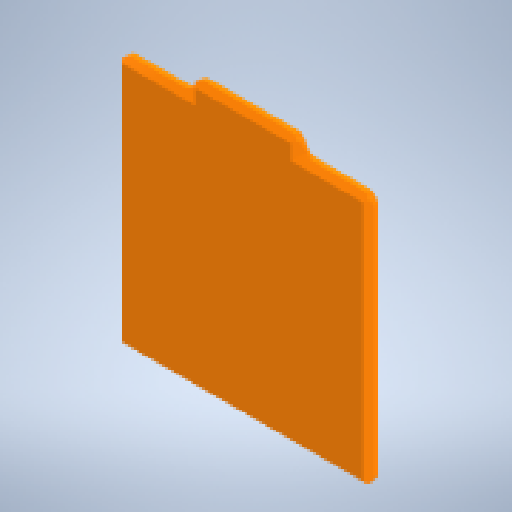
# Autodesk Inventor part: Lid
Saved by Autodesk Inventor 2025.1 (Build 291241000, 241)
## iProperties
Created: 2024-09-18
Part Number: Lid
Material: PET Plastic
Document SubType Name: Modeling
Designer: NDurn
Density: 1.541 g/cm^3
Appearance: Polycarbonate - Clear
Author: NDurn
Autodesk Inventor part; units mm, degrees
ref_plane "YZ Plane" through (0, 0, 0) normal (1, 0, 0) x (0, 1, 0)
ref_plane "XZ Plane" through (0, 0, 0) normal (0, 1, 0) x (-1, 0, 0)
ref_plane "XY Plane" through (0, 0, 0) normal (0, 0, 1) x (1, 0, 0)
sketch "Sketch1" plane through (0, 0, 0) normal (0, 0, 1) x (1, 0, 0)
  line L0 (37.5, -37.5) -> (-37.5, -37.5)
  line L1 (-37.5, -37.5) -> (-37.5, 37.5)
  line L2 (-37.5, 37.5) -> (37.5, 37.5)
  line L3 (37.5, 37.5) -> (37.5, -37.5)
  line L4 (37.5, -37.5) -> (-37.5, 37.5) construction
  line L5 (-37.5, -37.5) -> (37.5, 37.5) construction
  line L6 (32.5, 32.5) -> (-32.5, 32.5)
  line L7 (-32.5, 32.5) -> (-32.5, -32.5)
  line L8 (-32.5, -32.5) -> (32.5, -32.5)
  line L9 (32.5, -32.5) -> (32.5, 32.5)
  line L10 (32.5, 32.5) -> (-32.5, -32.5) construction
  line L11 (-32.5, 32.5) -> (32.5, -32.5) construction
  line L12 (30.5, 30.5) -> (-30.5, 30.5)
  line L13 (-30.5, 30.5) -> (-30.5, -30.5)
  line L14 (-30.5, -30.5) -> (30.5, -30.5)
  line L15 (30.5, -30.5) -> (30.5, 30.5)
  line L16 (30.5, 30.5) -> (-30.5, -30.5) construction
  line L17 (-30.5, 30.5) -> (30.5, -30.5) construction
  line L18 (-4.8636, 37.5) -> (-36.3868, 37.5)
  line L19 (0, 41.9833) -> (-15.7401, 41.9833)
  line L20 (-15.7401, 41.9833) -> (-15.7401, 37.5)
  line L21 (0, 41.9833) -> (15.8927, 41.9833)
  line L22 (15.8927, 41.9833) -> (15.8927, 37.5)
  point P0 (0, 0)
  dimension "d2" = 65
  dimension "d3" = 65
  dimension "d4" = 2
  dimension "d5" = 2
  dimension "d22" = 5
  dimension "d23" = 5
  constraints: 46 end point, 6 midpoint, 6 parallel, 5 horizontal, 5 perpendicular, 4 point on line
  measures "d2" distance of L8.end L7.end
  measures "d3" distance of L7.end L6.end
  measures "d4" distance between parallel lines of L8 L14
  measures "d5" distance between parallel lines of L7 L13
  measures "d22" distance between parallel lines of L2 L6
  measures "d23" distance between parallel lines of L7 L1
extrude "Extrusion1" add sketch "Sketch1" along normal blind 3 contours L0 L1 L2 L3 | L2 L20 L19 L21 L22 | L9 L8 L7 L6 | L15 L14 L13 L12
extrude "Extrusion2" add sketch "Sketch1" against normal blind 5 contours L9 L8 L7 L6
chamfer "Chamfer1" distance 1.5875 angle 45 8 edges at (0, -37.5, 3) (-37.5, 0, 3) (26.6963, 37.5, 3) (-26.62, 37.5, 3) (37.5, 0, 3) (15.8927, 39.7416, 3) (0.0763, 41.9833, 3) (-15.7401, 39.7416, 3)
fillet "Fillet2" radius 3.175 8 edges at (-37.5, -37.5, 0.7063) (37.5, -37.5, 0.7063) (37.5, 37.5, 0.7063) (-37.5, 37.5, 0.7063) (15.8927, 37.5, 0.7063) (15.8927, 41.9833, 0.7063) (-15.7401, 41.9833, 0.7063) (-15.7401, 37.5, 0.7063)
thicken "Thicken1" operation cut thickness 0.125 both sides no extend neighbours no toward (1, 0, 0) faces at (-32.5, 10.8333, -3.3333) (-10.8333, -32.5, -3.3333) (32.5, -10.8333, -3.3333) (10.8333, 32.5, -3.3333)
fillet "Fillet3" radius 1.5875 4 edges at (32.375, 0, -5) (-32.375, 0, -5) (0, 32.375, -5) (0, -32.375, -5)
body "Solid1"
